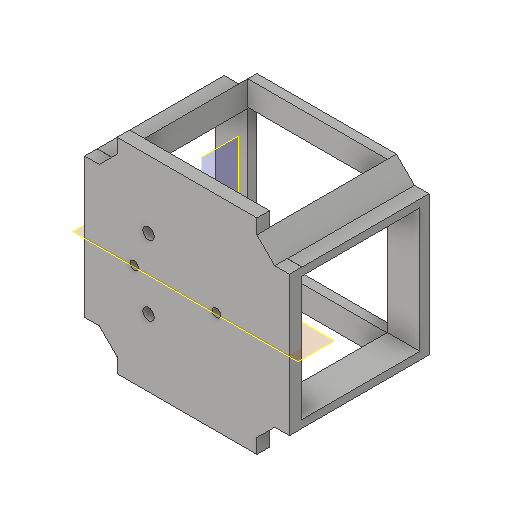
# Autodesk Inventor part: 20_Cube_Insert_Cube_Z-Stage_NEMA11_china_v3
Saved by Autodesk Inventor 2022 (Build 260153000, 153)
## iProperties
Created: 2019-07-01
Part Number: 20_Cube_Insert_Cube_Z-Stage_NEMA11_china_v3
Material: Generic
Document SubType Name: Modeling
Designer: diederichbenedict
Density: 1 g/cm^3
Appearance: Default
Author: diederichbenedict
Autodesk Inventor part; units mm, degrees
ref_plane "Work Plane1" through (-56.3599, 0, 22) normal (0, 0, -1) x (-1, 0, 0)
ref_plane "Arbeitsebene9" through (-61.2799, 5.9299, 18.95) normal (0, 0, 1) x (1, 0, 0)
sketch "Sketch1" plane through (-56.3599, 0, 22) normal (0, 0, -1) x (-1, 0, 0)
  line L0 (-4.0299, -0.3538) -> (-2.2322, 1.4439) construction
  arc A0 (-1.4439, 2.2322) -> (-2.2322, 1.4439) centre (-0.9299, 0.9299) ccw construction
  line L1 (-1.4439, 2.2322) -> (0.3538, 4.0299) construction
  line L2 (-37.8299, 42.8299) -> (-37.8299, 37.8299) construction
  line L3 (-37.8299, 37.8299) -> (-42.9208, 37.8299) construction
  line L4 (-37.8299, 42.2137) -> (-37.8299, 45.8299) construction
  line L5 (-37.8299, 45.8299) -> (-4.0299, 45.8299) construction
  line L6 (-4.0299, 45.8299) -> (-4.0299, 42.2137) construction
  line L7 (-4.0299, 4.0299) -> (0.3538, 4.0299) projected
  circle A1 centre (-20.9299, 20.9299) radius 17.5 projected
  line L8 (-20.9299, 58.9723) -> (17.1124, 20.9299) construction
  line L9 (17.1124, 20.9299) -> (-20.9299, -17.1124) construction
  line L10 (-20.9299, -17.1124) -> (-58.9723, 20.9299) construction
  line L11 (-58.9723, 20.9299) -> (-20.9299, 58.9723) construction
  line L12 (-20.9299, 58.9723) -> (-20.9299, -17.1124) construction
  line L13 (17.1124, 20.9299) -> (-58.9723, 20.9299) construction
  line L14 (-20.9299, 58.9723) -> (32.8701, 58.9723) construction
  line L15 (-43.4299, 43.4299) -> (1.5701, 43.4299) construction
  line L16 (1.5701, 43.4299) -> (1.5701, -1.5701) construction
  line L17 (1.5701, -1.5701) -> (-43.4299, -1.5701) construction
  line L18 (-43.4299, -1.5701) -> (-43.4299, 43.4299) construction
  line L19 (-43.4299, 43.4299) -> (1.5701, -1.5701) construction
  line L20 (1.5701, 43.4299) -> (-43.4299, -1.5701) construction
  line L21 (-43.4299, 5.3876) -> (-43.4299, 36.4723)
  line L22 (-43.4299, 36.4723) -> (-36.4723, 43.4299)
  line L23 (-36.4723, 43.4299) -> (-5.3876, 43.4299)
  line L24 (-5.3876, 43.4299) -> (1.5701, 36.4723)
  line L25 (1.5701, 36.4723) -> (1.5701, 5.3876)
  line L26 (1.5701, 5.3876) -> (-5.3876, -1.5701)
  line L27 (-5.3876, -1.5701) -> (-36.4723, -1.5701)
  line L28 (-36.4723, -1.5701) -> (-43.4299, 5.3876)
  line L29 (-4.0299, 42.2137) -> (-37.8299, 42.2137) projected
  line L30 (-4.0299, -0.3538) -> (-4.0299, 4.0299) projected
  circle A2 centre (-20.9299, 20.9299) radius 1.5
  line L31 (-10.9299, 10.9299) -> (-30.9299, 10.9299) construction
  line L32 (-30.9299, 10.9299) -> (-30.9299, 30.9299) construction
  line L33 (-30.9299, 30.9299) -> (-10.9299, 30.9299) construction
  line L34 (-10.9299, 30.9299) -> (-10.9299, 10.9299) construction
  line L35 (-10.9299, 10.9299) -> (-30.9299, 30.9299) construction
  line L36 (-30.9299, 10.9299) -> (-10.9299, 30.9299) construction
  circle A3 centre (-30.9299, 30.9299) radius 1.4
  circle A4 centre (-30.9299, 10.9299) radius 1.4
  circle A5 centre (-10.9299, 10.9299) radius 1.4
  line L37 (-45.8299, 37.8299) -> (-42.0723, 37.8299) construction
  line L38 (-42.1723, 37.7299) -> (-45.8299, 37.7299)
  line L39 (-45.8299, 37.7299) -> (-45.8299, 4.1299)
  line L40 (-45.8299, 4.1299) -> (-42.1723, 4.1299)
  line L41 (-42.1723, 4.1299) -> (-42.1723, 37.7299)
  line L42 (-45.8299, 4.0299) -> (-42.0723, 4.0299) construction
  line L43 (-45.8299, 37.8299) -> (-42.0723, 37.8299) projected
  line L44 (-37.7299, 45.8299) -> (-4.1299, 45.8299)
  line L45 (-4.1299, 45.8299) -> (-4.1299, 42.1723)
  line L46 (-4.1299, 42.1723) -> (-37.7299, 42.1723)
  line L47 (-37.7299, 42.1723) -> (-37.7299, 45.8299)
  line L48 (0.4701, 37.8299) -> (0.4701, 4.0299) construction
  line L49 (0.4701, 4.0299) -> (3.9701, 4.0299) construction
  line L50 (3.9701, 37.8299) -> (3.9701, 4.0299) construction
  line L51 (0.4701, 37.8299) -> (3.9701, 37.8299) construction
  line L52 (-45.8299, -3.9701) -> (-4.0299, -3.9701) construction
  line L53 (0.3124, 37.7299) -> (3.9701, 37.7299)
  line L54 (3.9701, 37.7299) -> (3.9701, 4.1299)
  line L55 (3.9701, 4.1299) -> (0.3124, 4.1299)
  line L56 (0.3124, 4.1299) -> (0.3124, 37.7299)
  line L57 (-4.1713, -0.3538) -> (-37.7299, -0.3538)
  line L58 (-37.7299, -0.3538) -> (-37.7299, -3.9701)
  line L59 (-37.7299, -3.9701) -> (-4.1713, -3.9701)
  line L60 (-4.1713, -3.9701) -> (-4.1713, -0.3538)
  point P0 (-37.8299, 4.0299)
  dimension "d18" = 53.8
  dimension "d19" = 45
  dimension "d20" = 53.8
  dimension "d21" = 45
  dimension "d22" = 45
  dimension "d30" = 20
  dimension "d31" = 20
  dimension "d32" = 2.8
  dimension "d33" = 2.8
  dimension "d34" = 2.8
  dimension "d35" = 3
  dimension "d36" = 0.1
  dimension "d37" = 0.1
  dimension "d38" = 0.1
  dimension "d39" = 0.1
  constraints: 86 end point, 21 point on line, 14 parallel, 8 perpendicular, 7 horizontal, 7 midpoint, 4 centre point, 4 coincident, 1 equal length
  measures "d18" distance of L8.start L8.end
  measures "d19" angle of L8 L14
  measures "d20" distance of L8.end L9.end
  measures "d21" distance of L16.end L17.end
  measures "d22" distance of L15.end L16.end
  measures "d30" distance of L32.end L33.end
  measures "d31" distance of L31.end L32.end
  measures "d32" diameter of A3
  measures "d33" diameter of A4
  measures "d34" diameter of A5
  measures "d35" diameter of A2
  measures "d36" distance between parallel lines of L38 L43
  measures "d37" distance between parallel lines of L40 L42
  measures "d38" distance between parallel lines of L45 L6
  measures "d39" distance between parallel lines of L4 L47
extrude "Extrusion1" add sketch "Sketch1" along normal up to surface (3.05 mm away) contours L30 L26 L57 L28 L41 L22 L46 L24 L56 L7 | L7 L26 L30 | L56 L24 L25 L26 | L26 L25 L24 L53 L54 L55 | L60 L59 L58 L57 L28 L27 L26 | L26 L27 L28 L57 | L46 L22 L29 L24 | L24 L29 L45 | L40 L39 L38 L22 L21 L28 | L28 L21 L22 L41 | L29 L22 L23 L24 | L24 L23 L22 L29 L47 L44 L45 | L47 L29 L22 | A1 | A2 | A3 | A4 | A5
sketch "Skizze4" plane through (-56.3599, 0, 18.95) normal (0, 0, -1) x (-1, 0, 0)
  line L0 (-37.7299, 42.1723) -> (-42.1723, 37.7299) projected
  line L1 (-42.1723, 37.7299) -> (-45.8299, 37.7299) projected
  line L2 (-45.8299, 37.7299) -> (-45.8299, 4.1299) construction
  line L3 (-45.8299, 4.1299) -> (-42.1723, 4.1299) projected
  line L4 (-42.1723, 4.1299) -> (-37.6885, -0.3538) projected
  line L5 (-37.6885, -0.3538) -> (-37.7299, -0.3538) projected
  line L6 (-37.7299, -0.3538) -> (-37.7299, -3.9701) projected
  line L7 (-37.7299, -3.9701) -> (-4.1713, -3.9701) construction
  line L8 (-4.1713, -3.9701) -> (-4.1713, -0.3538) projected
  line L9 (-4.1713, -0.3538) -> (0.3124, 4.1299) projected
  line L10 (0.3124, 4.1299) -> (3.9701, 4.1299) projected
  line L11 (3.9701, 4.1299) -> (3.9701, 37.7299) construction
  line L12 (3.9701, 37.7299) -> (0.3124, 37.7299) projected
  line L13 (0.3124, 37.7299) -> (-4.1299, 42.1723) projected
  line L14 (-4.1299, 42.1723) -> (-4.1299, 45.8299) projected
  line L15 (-4.1299, 45.8299) -> (-37.7299, 45.8299) construction
  line L16 (-37.7299, 45.8299) -> (-37.7299, 42.1723) projected
  line L17 (-37.9299, 46.0299) -> (-3.9299, 46.0299) construction
  line L18 (-3.9299, 46.0299) -> (-3.9299, 42.2551)
  line L19 (-3.9299, 42.2551) -> (0.3953, 37.9299)
  line L20 (0.3953, 37.9299) -> (4.1701, 37.9299)
  line L21 (4.1701, 37.9299) -> (4.1701, 3.9299) construction
  line L22 (4.1701, 3.9299) -> (0.3953, 3.9299)
  line L23 (0.3953, 3.9299) -> (-3.9713, -0.4367)
  line L24 (-3.9713, -0.4367) -> (-3.9713, -4.1701)
  line L25 (-3.9713, -4.1701) -> (-37.9299, -4.1701) construction
  line L26 (-37.9299, -4.1701) -> (-37.9299, -0.3953)
  line L27 (-37.9299, -0.3953) -> (-42.2551, 3.9299)
  line L28 (-42.2551, 3.9299) -> (-46.0299, 3.9299)
  line L29 (-46.0299, 3.9299) -> (-46.0299, 37.9299) construction
  line L30 (-46.0299, 37.9299) -> (-42.2551, 37.9299)
  line L31 (-42.2551, 37.9299) -> (-37.9299, 42.2551)
  line L32 (-37.9299, 42.2551) -> (-37.9299, 46.0299)
  line L33 (-45.8299, 37.7299) -> (-45.8299, 37.9299)
  line L34 (-4.1299, 45.8299) -> (-37.7299, 45.8299) projected
  line L35 (-37.7299, 45.8299) -> (-37.9299, 45.8299)
  line L36 (-4.1299, 45.8299) -> (-3.9299, 45.8299)
  line L37 (3.9701, 37.7299) -> (3.9701, 37.9299)
  line L38 (3.9701, 4.1299) -> (3.9701, 37.7299) projected
  line L39 (3.9701, 4.1299) -> (3.9701, 3.9299)
  line L40 (-4.1713, -3.9701) -> (-3.9713, -3.9701)
  line L41 (-37.7299, -3.9701) -> (-37.9299, -3.9701)
  line L42 (-45.8299, 4.1299) -> (-45.8299, 3.9299)
  point P0 (-56.3599, 0)
  dimension "d40" = 0.2
  constraints: 48 end point, 12 point on line, 4 perpendicular, 15 other
  measures "d40" distance between parallel lines of L15 L17
extrude "IM_offset" add sketch "Skizze4" against normal up to surface (3.05 mm away)
ref_plane "Arbeitsebene5" through (-35.4299, 3.9299, 22) normal (-1, 0, 0) x (0, 0, 1)
ref_plane "Arbeitsebene6" through (-18.4299, 20.9299, 22) normal (0, 1, 0) x (-1, 0, 0)
sketch "Skizze31" plane through (-10.5299, 3.9299, 18.95) normal (1, 0, 0) x (0, 0, -1)
  line L0 (0, 0) -> (0, 34) projected
  line L1 (0, 34) -> (-3.05, 34) projected
  line L2 (-3.05, 0) -> (-3.05, 34) projected
  line L3 (0, 0) -> (-3.05, 0) projected
  line L4 (-3.05, -5.85) -> (-10.55, -5.85) projected
  line L5 (-3.05, 33.97) -> (-3.05, -5.85) projected
  line L6 (-3.05, 33.97) -> (31.05, 33.97) projected
  line L7 (31.05, 39.85) -> (31.05, 33.97) projected
  line L8 (-10.55, 39.85) -> (31.05, 39.85) projected
  line L9 (-10.55, -5.85) -> (-10.55, 39.85) projected
  line L10 (31.05, 39.85) -> (38.55, 39.85) projected
  line L11 (31.05, 0.03) -> (31.05, 39.85) projected
  line L12 (31.05, 0.03) -> (-3.05, 0.03) projected
  line L13 (-3.05, -5.85) -> (-3.05, 0.03) projected
  line L14 (38.55, -5.85) -> (-3.05, -5.85) projected
  line L15 (38.55, 39.85) -> (38.55, -5.85) projected
  line L16 (0, 0) -> (0, 34) projected
  line L17 (0, 33.97) -> (30.9, 33.97)
  line L18 (30.9, 33.97) -> (30.9, 32.1075)
  line L19 (30.9, 32.1075) -> (0, 32.1075)
  line L20 (0, 32.1075) -> (0, 33.97)
  line L21 (30.9, 1.8846) -> (0, 1.8846)
  line L22 (0, 1.8846) -> (0, 0.03)
  line L23 (0, 0.03) -> (30.9, 0.03)
  line L24 (30.9, 0.03) -> (30.9, 1.8846)
  circle A0 centre (20.35, 17) radius 6.5 projected
  line L25 (30.9, 32.1075) -> (30.9, 1.8846)
  line L26 (28.5, 2) -> (28.5, 32) projected
  line L27 (28.7, 32.1075) -> (28.7, 1.8846)
  point P0 (18.95, -3.9299)
  point P1 (0, 33.97)
  point P2 (0, 1.8846)
  point P3 (0, 0.03)
  dimension "d181" = 0
  dimension "d182" = 0
  dimension "d183" = 0.15
  dimension "d184" = 0.2
  constraints: 20 end point, 5 point on line, 4 parallel, 3 perpendicular, 2 horizontal, 1 vertical
  measures "d181" distance between parallel lines of L23 L12
  measures "d182" distance between parallel lines of L6 L17
  measures "d183" distance between parallel lines of L18 L11
  measures "d184" distance between parallel lines of L27 L26
ref_plane "Arbeitsebene10" through (-18.4599, -3.9201, -16.28) normal (-1, 0, 0) x (0, 0, 1)
extrude "Extrusion26" add sketch "Skizze31" against normal up to surface (7.93 mm away) contours L0 L21 L24 L12 | L0 L6 L18 L19 | L27 L19 L25 L21
sketch "Skizze32" plane through (-10.5299, 3.9599, -11.95) normal (0, 0, -1) x (-1, 0, 0)
  line L0 (0, 0) -> (0, 33.94) projected
  line L1 (0, 33.94) -> (7.93, 33.94) projected
  line L2 (0, 0) -> (7.93, 0) projected
  line L3 (7.9, -4.3552) -> (3.5748, -0.03) construction
  line L4 (4.3761, 34.7834) -> (7.1197, 37.7973) construction
  line L5 (7.9, 38.2952) -> (3.5748, 33.97) construction
  line L6 (3.5448, 33.94) -> (7.93, 38.3252)
  line L7 (7.93, 38.3252) -> (7.93, 33.94)
  line L8 (7.93, 1.8546) -> (7.93, 0) projected
  line L9 (7.93, 0) -> (7.93, -0.13)
  line L10 (3.5448, 0) -> (7.8, -4.2552)
  line L11 (7.8, -4.2552) -> (7.8, 0)
  point P0 (-10.5299, -3.9599)
  dimension "d187" = 45
  dimension "d188" = 0
  dimension "d189" = 0
  constraints: 10 end point, 4 point on line, 2 collinear, 2 vertical, 3 other
  measures "d188" distance between parallel lines of L10 L3
  measures "d189" distance between parallel lines of L5 L6
extrude "Extrusion27" add sketch "Skizze32" against normal up to surface (30.9 mm away)
mirror "Spiegeln2" about plane through (-35.4299, 3.9299, 22) normal (-1, 0, 0) of "Extrusion26", "Extrusion27"
sketch "Skizze33" plane through (-10.5299, 3.9599, -11.95) normal (0, 0, -1) x (-1, 0, 0)
  line L0 (0.05, 39.82) -> (0.05, -5.88) projected
  line L1 (41.87, 0) -> (41.87, 38.3252) projected
  line L2 (7.93, 0) -> (7.93, 38.3252) projected
  line L3 (41.87, 38.3252) -> (7.93, 38.3252)
  line L4 (7.93, 38.3252) -> (7.93, 32.3252)
  line L5 (7.93, 32.3252) -> (41.87, 32.3252)
  line L6 (41.87, 32.3252) -> (41.87, 38.3252)
  line L7 (46.2552, 0) -> (42, -4.2552) projected
  line L8 (42, -4.2552) -> (7.93, -4.2552)
  line L9 (7.93, -4.2552) -> (7.93, 1.7448)
  line L10 (7.93, 1.7448) -> (42, 1.7448)
  line L11 (42, 1.7448) -> (42, -4.2552)
  point P0 (-10.5299, -3.9599)
  point P1 (7.93, 38.3252)
  point P2 (41.87, 32.3252)
  dimension "d192" = 6
  dimension "d193" = 6
  constraints: 16 end point, 4 parallel, 2 horizontal, 2 perpendicular, 2 point on line
  measures "d192" distance of L4.end L3.end
  measures "d193" distance of L8.end L9.end
extrude "Extrusion28" add sketch "Skizze33" against normal up to surface (2.2 mm away) contours L5 L2 L3 L1 | L10 L11 L8 L9 L2
sketch "Skizze34" plane through (-56.3599, 0, 22) normal (0, 0, 1) x (1, 0, 0)
  line L0 (-4.9201, 35.9299) -> (-4.9201, 5.9299) projected
  line L1 (83.0799, 5.9299) -> (-4.9201, 5.9299) projected
  line L2 (83.0799, 35.9299) -> (83.0799, 5.9299) projected
  line L3 (83.0799, 35.9299) -> (-4.9201, 35.9299) projected
  circle A0 centre (8.0799, 20.9299) radius 1.025 projected
  circle A1 centre (28.0799, 20.9299) radius 1.025 projected
  circle A2 centre (48.0799, 20.9299) radius 1.025 projected
  circle A3 centre (68.0799, 20.9299) radius 1.025 projected
  circle A4 centre (66.5799, 29.4299) radius 1.7 projected
  circle A5 centre (66.5799, 12.4299) radius 1.7 projected
  circle A6 centre (11.5799, 12.4299) radius 1.7 construction
  circle A7 centre (11.5799, 29.4299) radius 1.7 construction
  circle A8 centre (11.5799, 12.4299) radius 1.4
  circle A9 centre (11.5799, 29.4299) radius 1.4
  point P0 (56.3599, 0)
  dimension "d198" = 2.8
  dimension "d199" = 2.8
  constraints: 2 centre point, 2 coincident
  measures "d198" diameter of A8
  measures "d199" diameter of A9
extrude "Extrusion29" cut sketch "Skizze34" against normal blind 10 contours A0 | A1 | A8 | A9
body "Solid1"
